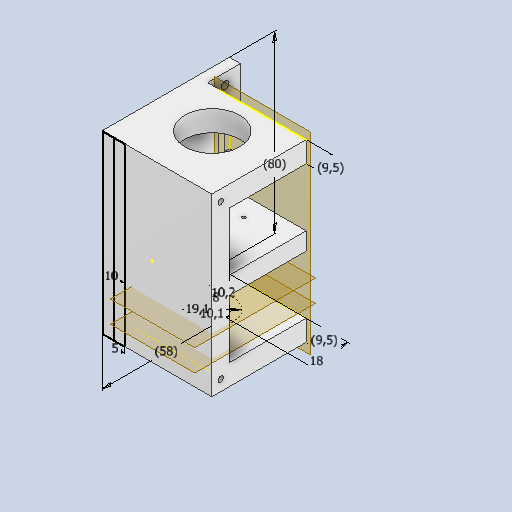
# Autodesk Inventor part: daVinci_Head_Sensorpart
Saved by Autodesk Inventor 2024 (Build 280153000, 153)
## iProperties
Created: 2022-10-05
Part Number: daVinci_Head_Sensorpart
Material: PBT-Kunststoff
Document SubType Name: Modeling
Designer: alexw
Density: 1.31 g/cm^3
Appearance: Glatt - Weiß
Mass: 163.908 g
Surface Area: 302.501 cm^2
Volume: 125.121 cm^3
SensorBox_Width: 58,000 mm
SensorBox_Length: 80,000 mm
Author: alexw
Autodesk Inventor part; units mm, degrees
ref_plane "YZ Plane" through (0, 0, 0) normal (1, 0, 0) x (0, 1, 0)
ref_plane "XZ Plane" through (0, 0, 0) normal (0, 1, 0) x (-1, 0, 0)
ref_plane "XY Plane" through (0, 0, 0) normal (0, 0, 1) x (1, 0, 0)
ref_plane "Arbeitsebene1" through (0, 0, 0) normal (0, 0, 1) x (1, 0, 0)
sketch "Skizze1" plane through (0, 0, 0) normal (0, 0, 1) x (1, 0, 0)
  line L0 (-10.5, 20.2) -> (-8, 20.2) projected
  line L1 (-8, 20.2) -> (-8, 30.5) projected
  line L2 (-8, 30.5) -> (-2.5, 30.5) projected
  line L3 (-2.5, 30.5) -> (-2.5, 34.5) projected
  line L4 (-2.5, 34.5) -> (8, 34.5) projected
  line L5 (8, 34.5) -> (8, 30.5) projected
  line L6 (8, 30.5) -> (27, 30.5) projected
  line L7 (27, 30.5) -> (27, 40) projected
  line L8 (27, 40) -> (-13, 40) projected
  line L9 (-13, -40) -> (-13, 40) projected
  line L10 (27, -40) -> (-13, -40) projected
  line L11 (27, -40) -> (27, -30.5) projected
  line L12 (27, -30.5) -> (8, -30.5) projected
  line L13 (8, -30.5) -> (8, -34.5) projected
  line L14 (8, -34.5) -> (-2.5, -34.5) projected
  line L15 (-2.5, -34.5) -> (-2.5, -30.5) projected
  line L16 (-2.5, -30.5) -> (-8, -30.5) projected
  line L17 (-8, -30.5) -> (-8, -2) projected
  line L18 (-8, -2) -> (-1, -2) projected
  line L19 (-1, -2) -> (-1, 2) projected
  line L20 (-1, 2) -> (-8, 2) projected
  line L21 (-8, 2) -> (-8, 14.2) projected
  line L22 (-8, 14.2) -> (-10.5, 14.2) projected
  line L23 (-10.5, 20.2) -> (-10.5, 14.2) projected
  line L24 (8, 30.5) -> (-2.5, 30.5)
  line L25 (8, -30.5) -> (-2.5, -30.5)
  line L26 (-8, -2) -> (-8, 2)
  line L27 (-8, 14.2) -> (-8, 20.2)
  point P0 (0, 0)
  constraints: 8 end point, 2 collinear, 1 horizontal, 1 perpendicular
ref_plane "Arbeitsebene2" through (0, 0, 0) normal (0, 0, 1) x (1, 0, 0)
extrude "Extrusion1" add sketch "Skizze1" along normal blind 43 contours L23 L22 L21 L26 L17 L16 L15 L14 L13 L12 L11 L10 L9 L8 L7 L6 L5 L4 L3 L2 L1 L0 | L0 L27 L22 L23 | L3 L4 L5 L24 | L25 L13 L14 L15
sketch "Skizze2" plane through (-8, -30.5, 0) normal (0, 1, 0) x (1, 0, 0)
  circle A0 centre (10.2, -18) radius 9.55 construction
  line L0 (0, 0) -> (0, -43) construction
  line L1 (35, -43) -> (0, -43) construction
  circle A1 centre (10.2, -18) radius 5.05
  circle A2 centre (10.2, -18) radius 4
  point P0 (8, 0)
  dimension "d2" = 19.1
  dimension "d18" = 10.1
  dimension "d62" = 10.2
  dimension "d63" = 18
  dimension "d64" = 8
  constraints: 3 centre point, 1 coincident, 1 concentric
  measures "d2" diameter of A0
  measures "d18" diameter of A1
  measures "d62" distance from line of L0 A0.centre
  measures "d63" vertical distance of L0.start A0.centre
  measures "d64" diameter of A2
sketch "Sketch9" plane through (0, 0, 0) normal (0, 0, -1) x (-1, 0, 0)
  line L0 (-27, 40) -> (13, 40) projected
  line L1 (8, 30.5) -> (-27, 30.5) projected
  line L2 (-27, -30.5) -> (8, -30.5) projected
  line L3 (13, -40) -> (-27, -40) projected
  point P0 (0, 0)
  dimension "d67" = 9.5
  dimension "d68" = 9.5
  measures "d67" distance between parallel lines of L0 L1
  measures "d68" distance between parallel lines of L2 L3
extrude "Extrusion2" cut sketch "Skizze2" along normal through all both and the other way through all contours A1 | A2
ref_plane "Arbeitsebene4" through (-8, -15, 0) normal (0, 1, 0) x (1, 0, 0)
sketch "Skizze3" plane through (-13, -30.5, 0) normal (0, -1, 0) x (1, 0, 0)
  circle A0 centre (15.2, 18) radius 9.525 construction
  line L0 (15.2, 27.525) -> (15.2, 8.475) construction
  circle A1 centre (15.2, 18) radius 10.45 construction
  line L1 (15.2, 18) -> (4.75, 18) construction
  point P0 (13, 0)
  point P1 (20.425, 8.95)
  point P2 (20.425, 27.05)
  dimension "d57" = 20.9
  dimension "d10" = 19.05
  dimension "d60" = 360
  constraints: 4 end point, 3 coincident, 2 midpoint, 2 point on circle, 1 centre point, 1 horizontal, 1 horizontal alignment, 1 vertical, 6 other
  measures "d10" diameter of A0
ref_plane "Arbeitsebene3" through (-8, -25, 0) normal (0, 1, 0) x (1, 0, 0)
sketch "Skizze4" plane through (-8, -30.5, 0) normal (1, 0, 0) x (0, 0, -1)
  line L0 (-43, 70.5) -> (-43, -9.5) construction
  line L1 (0, 70.5) -> (0, -9.5) construction
  line L2 (-43, 34.5) -> (0, 34.5)
  line L3 (0, 34.5) -> (0, 26.5)
  line L4 (0, 26.5) -> (-43, 26.5)
  line L5 (-43, 26.5) -> (-43, 34.5)
  line L6 (0, 0) -> (-43, 0) projected
  line L7 (-54.6, 15.5) -> (26.6, 15.5) construction
  line L8 (-43, 61) -> (-43, 70.5) projected
  line L9 (0, 0) -> (-43, 0) projected
  line L10 (-43, 61) -> (-35, 61)
  line L11 (-35, 61) -> (-35, 0)
  line L12 (-35, 0) -> (-43, 0)
  line L13 (-43, 0) -> (-43, 61)
  point P0 (0, 30.5)
  point P1 (-43, 26.5)
  point P2 (-43, 0)
  point P3 (-35, 0)
  point P4 (-35, 26.5)
  point P5 (-35, 34.5)
  point P6 (-43, 30.5)
  dimension "d13" = 8
  dimension "d36" = 8
  constraints: 16 end point, 4 parallel, 3 point on line, 2 horizontal, 2 midpoint, 2 perpendicular
  measures "d13" distance between parallel lines of L4 L2
  measures "d36" distance between parallel lines of L13 L11
extrude "Extrusion3" add sketch "Skizze4" along normal up to surface (35 mm away)
extrude "Extrusion4" cut sketch "Skizze2" along normal through all contours A1 | A2
extrude "Extrusion5" cut sketch "Skizze2" against normal blind 4 from surface at 0 contours A1 | A2
extrude "Extrusion6" cut sketch "Skizze2" along normal blind 4 from surface at 26.5 contours A1 | A2
hole "Bohrung1" at (-8.25, -30.5, 18) at (7.425, -30.5, 8.95) at (7.425, -30.5, 27.05) direction (0, 1, 0) diameter 1.567 depth 34.5 tip angle 118 thread size "M2x0.4" class "6H" standard "ISO Metric profile"
sketch "Skizze5" plane through (0, 0, 43) normal (0, 0, 1) x (1, 0, 0)
  line L0 (-13, 40) -> (-13, -40) projected
  line L1 (-13, 40) -> (-23, 40)
  line L2 (-23, 40) -> (-23, -40)
  line L3 (-23, -40) -> (-13, -40)
  line L4 (-13, -40) -> (-13, 40)
  line L5 (-18, 40) -> (-18, -40)
  point P0 (0, 0)
  dimension "d30" = 10
  dimension "d31" = 5
  constraints: 10 end point, 2 midpoint, 2 parallel, 2 perpendicular, 1 horizontal, 1 point on line
  measures "d30" distance between parallel lines of L0 L2
  measures "d31" distance between parallel lines of L0 L5
extrude "Extrusion7" add sketch "Skizze5" against normal up to surface (43 mm away)
extrude "Extrusion8" add sketch "Skizze5" against normal blind 15 from surface at -43 contours L5 L3 L2 L1
sketch "Skizze6" plane through (-18, -40, -15) normal (1, 0, 0) x (0, 0, -1)
  line L0 (-7, 75) -> (-7, 5) construction
  line L1 (-7, 40) -> (0, 40) construction
  line L2 (0, 80) -> (0, 0) construction
  line L3 (-15, -16) -> (-15, 96) construction
  point P0 (-15, 40)
  dimension "d37" = 8
  dimension "d38" = 5
  constraints: 4 end point, 2 coincident, 2 midpoint, 1 horizontal, 1 vertical
  measures "d37" distance between parallel lines of L0 L3
  measures "d38" vertical distance of L2.start point (-7, 75)
hole "Bohrung2" at (-18, -35, -8) at (-18, 35, -8) direction (-1, 0, 0) diameter 3.4 end through all clearance for "Inbusschraube DIN EN ISO 4762" size "M3" standard "DIN"
sketch "Sketch14" plane through (-18, 4, 35) normal (1, 0, 0) x (0, 0, -1)
  line L0 (-8, 36) -> (50, 36) projected
  line L1 (-8, -44) -> (50, -44) projected
  line L2 (50, 36) -> (35, 36)
  line L3 (35, 36) -> (35, -44)
  line L4 (35, -44) -> (50, -44)
  line L5 (50, -44) -> (50, 36)
  line L6 (35, -44) -> (35, -34.5) projected
  circle A0 centre (43, 31) radius 1.7 projected
  circle A1 centre (43, -39) radius 1.7 projected
  point P0 (35, -4)
  constraints: 8 end point, 2 parallel, 1 collinear, 1 horizontal, 1 perpendicular, 1 point on line
sketch "Skizze7" plane through (-23, -40, 43) normal (-1, 0, 0) x (0, 0, 1)
  line L0 (-58, 0) -> (-58, 80) projected
  line L1 (0, 80) -> (0, 0) projected
  point P0 (-43, 40)
  dimension "SensorBox_Width" = 58
  dimension "SensorBox_Length" = 80
  measures "SensorBox_Width" distance between parallel lines of L0 L1
  measures "SensorBox_Length" distance of L0.start L0.end
sketch "Skizze8" plane through (27, -40, 0) normal (1, 0, 0) x (0, 0, -1)
  line L0 (-39, 5) -> (-39, 75) construction
  line L1 (-43, 0) -> (-43, 80) construction
  line L2 (-43, 40) -> (-39, 40) construction
  point P0 (0, 40)
  dimension "d48" = 4
  dimension "d49" = 70
  constraints: 4 end point, 2 midpoint, 1 horizontal, 1 vertical
  measures "d48" distance between parallel lines of L1 L0
  measures "d49" distance of L0.start L0.end
hole "Bohrung3" at (27, 35, 39) at (27, -35, 39) direction (-1, 0, 0) diameter 2.459 depth 12 tip angle 118 thread size "M3x0.5" class "6H" standard "ISO Metric profile"
extrude "Extrusion9" add sketch "Skizze2" along normal blind 5.5 from surface at -9.5
sketch "Sketch10" plane through (-8, 4, 0) normal (1, 0, 0) x (0, 0, -1)
  spline S0 degree 2 poles (-18.7425, 0) (-18, 0.4228) (-17.2575, 0) knots 0 0 0 1 1 1 weights 1 3.134 1 projected
  line L0 (-17.2575, 0) -> (0, 0) projected
  line L1 (0, 0) -> (0, 26.5) projected
  line L2 (0, 26.5) -> (-35, 26.5) projected
  line L3 (-35, 26.5) -> (-35, 0) projected
  line L4 (-35, 0) -> (-18.7425, 0) projected
  line L5 (0, -34.5) -> (0, -8) projected
  line L6 (-18.7425, -34.5) -> (-35, -34.5) projected
  line L7 (0, -8) -> (-35, -8)
  line L8 (-35, -8) -> (-35, -34.5)
  line L9 (-35, -34.5) -> (0, -34.5)
  line L10 (0, -34.5) -> (0, -8)
  point P0 (0, -4)
  point P1 (0, -34.5)
  constraints: 8 end point, 2 parallel, 1 horizontal, 1 horizontal alignment, 1 perpendicular
extrude "Extrusion10" cut sketch "Sketch10" against normal up to surface (10 mm away)
delete faces "Delete Face1" heal yes whole lump no faces at (-13.25, 4.2311, 18.3108)
extrude "Extrusion11" add sketch "Skizze2" along normal blind 5 from surface at 26.5
sketch "Sketch11" plane through (27, 40, 43) normal (0, 1, 0) x (1, 0, 0)
  circle A0 centre (-24.8, 25) radius 5.05 projected
  circle A1 centre (-24.8, 25) radius 12.5
  point P0 (-27, 43)
  dimension "d73" = 25
  constraints: 1 centre point, 1 coincident
  measures "d73" diameter of A1
extrude "Extrusion12" cut sketch "Sketch11" against normal up to surface (9.5 mm away)
sketch "Sketch12" plane through (27, -40, 0) normal (0, -1, 0) x (1, 0, 0)
  circle A0 centre (-24.8, 18) radius 4 projected
  point P0 (-27, 0)
extrude "Extrusion13" add sketch "Sketch12" against normal blind 2
sketch "Sketch13" plane through (-18, 4, 35) normal (0, 1, 0) x (1, 0, 0)
  line L0 (0, 50) -> (0, 35) projected
  line L1 (0, 50) -> (-5, 50) projected
  line L2 (-4, 46.9282) -> (0, 40)
  line L3 (-4, 46.9282) -> (-5, 46.9282)
  line L4 (-5, -8) -> (-5, 50) projected
  line L5 (-5, 50) -> (-5, 46.9282)
  point P0 (18, 35)
  dimension "d82" = 10
  dimension "d83" = 30
  dimension "d84" = 1
  constraints: 6 end point, 2 point on line, 1 horizontal, 1 perpendicular
  measures "d82" distance of L0.start L2.end
  measures "d83" angle of L0 L2
  measures "d84" distance from line of L4 L2.start
extrude "Extrusion14" cut sketch "Sketch13" along normal blind 18.3
equation "\"d36\" = d13"
body "Solid2"
